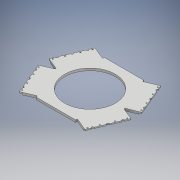
# Autodesk Inventor part: topplate change axes
Saved by Autodesk Inventor 2018 (Build 220112000, 112)
## iProperties
Created: 2018-06-04
Part Number: topplate change axes
Material: Generic
Document SubType Name: Modeling
Designer: John Viljoen
Density: 1 g/cm^3
Appearance: Default
Author: John Viljoen
Autodesk Inventor part; units mm, degrees
ref_plane "YZ Plane" through (0, 0, 0) normal (1, 0, 0) x (0, 1, 0)
ref_plane "XZ Plane" through (0, 0, 0) normal (0, 1, 0) x (-1, 0, 0)
ref_plane "XY Plane" through (0, 0, 0) normal (0, 0, 1) x (1, 0, 0)
sketch "Sketch1" plane through (0, 0, 0) normal (0, 0, 1) x (1, 0, 0)
  line L0 (0, 5) -> (0, 0)
  line L1 (0, 0) -> (109.5, 0)
  line L2 (109.5, 0) -> (109.5, 5)
  line L3 (109.5, 5) -> (145.4775, -9.976)
  line L4 (145.4775, -9.976) -> (150.4727, 2.0242)
  arc A0 (152.913, 7.8866) -> (150.4727, 2.0242) centre (151.6928, 4.9554) ccw
  line L5 (152.913, 7.8866) -> (162.9034, 31.887)
  arc A1 (165.3436, 37.7494) -> (162.9034, 31.887) centre (164.1235, 34.8182) ccw
  line L6 (165.3436, 37.7494) -> (175.334, 61.7498)
  arc A2 (177.7743, 67.6121) -> (175.334, 61.7498) centre (176.5542, 64.6809) ccw
  line L7 (177.7743, 67.6121) -> (182.7695, 79.6123)
  line L8 (182.7695, 79.6123) -> (146.792, 94.5883)
  line L9 (146.792, 94.5883) -> (182.7695, 109.5643)
  line L10 (182.7695, 109.5643) -> (177.7743, 121.5645)
  arc A3 (175.334, 127.4269) -> (177.7743, 121.5645) centre (176.5542, 124.4957) ccw
  line L11 (175.334, 127.4269) -> (165.3436, 151.4273)
  arc A4 (162.9034, 157.2897) -> (165.3436, 151.4273) centre (164.1235, 154.3585) ccw
  line L12 (162.9034, 157.2897) -> (152.913, 181.29)
  arc A5 (150.4727, 187.1524) -> (152.913, 181.29) centre (151.6928, 184.2212) ccw
  line L13 (150.4727, 187.1524) -> (145.4775, 199.1526)
  line L14 (145.4775, 199.1526) -> (109.5, 184.1766)
  line L15 (109.5, 184.1766) -> (109.5, 189.1766)
  line L16 (109.5, 189.1766) -> (0, 189.1766)
  line L17 (0, 189.1766) -> (0, 184.1766)
  line L18 (0, 184.1766) -> (-35.9775, 199.1526)
  line L19 (-35.9775, 199.1526) -> (-40.9727, 187.1524)
  arc A6 (-43.413, 181.29) -> (-40.9727, 187.1524) centre (-42.1928, 184.2212) ccw
  line L20 (-43.413, 181.29) -> (-53.4034, 157.2897)
  arc A7 (-55.8436, 151.4273) -> (-53.4034, 157.2897) centre (-54.6235, 154.3585) ccw
  line L21 (-55.8436, 151.4273) -> (-65.834, 127.4269)
  arc A8 (-68.2743, 121.5645) -> (-65.834, 127.4269) centre (-67.0542, 124.4957) ccw
  line L22 (-68.2743, 121.5645) -> (-73.2695, 109.5643)
  line L23 (-73.2695, 109.5643) -> (-37.292, 94.5883)
  line L24 (-37.292, 94.5883) -> (-73.2695, 79.6123)
  line L25 (-73.2695, 79.6123) -> (-68.2743, 67.6121)
  arc A9 (-65.834, 61.7498) -> (-68.2743, 67.6121) centre (-67.0542, 64.6809) ccw
  line L26 (-65.834, 61.7498) -> (-55.8436, 37.7494)
  arc A10 (-53.4034, 31.887) -> (-55.8436, 37.7494) centre (-54.6235, 34.8182) ccw
  line L27 (-53.4034, 31.887) -> (-43.413, 7.8866)
  arc A11 (-40.9727, 2.0242) -> (-43.413, 7.8866) centre (-42.1928, 4.9554) ccw
  line L28 (-40.9727, 2.0242) -> (-35.9775, -9.976)
  line L29 (-35.9775, -9.976) -> (0, 5)
  circle A12 centre (-35.5423, -2.7596) radius 1.5
  circle A13 centre (54.75, 94.5883) radius 70
  circle A14 centre (154.973, 168.0663) radius 1.5
  circle A15 centre (-67.8404, 114.345) radius 1.5
  circle A16 centre (-57.907, 138.2085) radius 1.5
  circle A17 centre (-45.4757, 168.0728) radius 1.5
  circle A18 centre (-35.5423, 191.9362) radius 1.5
  circle A19 centre (145.0396, 191.9297) radius 1.5
  circle A20 centre (167.4043, 138.2019) radius 1.5
  circle A21 centre (177.3377, 114.3385) radius 1.5
  circle A22 centre (177.3404, 74.8316) radius 1.5
  circle A23 centre (167.407, 50.9682) radius 1.5
  circle A24 centre (154.9757, 21.1038) radius 1.5
  circle A25 centre (145.0423, -2.7596) radius 1.5
  circle A26 centre (-67.8404, 74.8316) radius 1.5
  circle A27 centre (-57.907, 50.9682) radius 1.5
  circle A28 centre (-45.4757, 21.1038) radius 1.5
  constraints: 60 end point, 29 centre point, 24 point on circle
extrude "Extrusion1" add sketch "Sketch1" along normal blind 6.35
sketch "Sketch2" plane through (-35.9775, 199.1526, 6.35) normal (0.3842953, 0.9232102, 0) x (0.9232102, -0.3842953, 0)
  line L0 (0, 6.35) -> (6.35, 6.35)
  line L1 (6.35, 6.35) -> (6.35, 3.175)
  line L2 (6.35, 3.175) -> (0, 3.175)
  line L3 (0, 3.175) -> (0, 6.35)
  point P0 (109.7482, 6.35)
  dimension "d2" = 6.35
  constraints: 8 end point, 2 parallel, 1 horizontal, 1 perpendicular
  measures "d2" distance of L1.end L2.end
extrude "Extrusion2" cut sketch "Sketch2" against normal through all
sketch "Sketch3" plane through (-73.2695, 79.6123, 6.35) normal (-0.3842953, 0.9232102, 0) x (0.9232102, 0.3842953, 0)
  line L0 (0, 6.35) -> (6.35, 6.35)
  line L1 (6.35, 6.35) -> (6.35, 3.175)
  line L2 (6.35, 3.175) -> (0, 3.175)
  line L3 (0, 3.175) -> (0, 6.35)
  point P0 (37.0485, 6.35)
  dimension "d5" = 6.35
  constraints: 8 end point, 2 parallel, 1 horizontal, 1 perpendicular
  measures "d5" distance of L1.end L2.end
extrude "Extrusion3" cut sketch "Sketch3" against normal through all
sketch "Sketch4" plane through (109.5, 184.1766, 6.35) normal (-0.3842953, 0.9232102, 0) x (0.9232102, 0.3842953, 0)
  line L0 (38.97, 6.35) -> (32.62, 6.35)
  line L1 (32.62, 6.35) -> (32.62, 3.175)
  line L2 (32.62, 3.175) -> (38.97, 3.175)
  line L3 (38.97, 3.175) -> (38.97, 6.35)
  point P0 (-171.8697, 6.35)
  dimension "d8" = 6.35
  constraints: 8 end point, 2 parallel, 1 horizontal, 1 perpendicular
  measures "d8" distance of L2.end L1.end
extrude "Extrusion4" cut sketch "Sketch4" against normal through all
sketch "Sketch5" plane through (146.792, 94.5883, 6.35) normal (0.3842953, 0.9232102, 0) x (0.9232102, -0.3842953, 0)
  line L0 (38.97, 6.35) -> (32.62, 6.35)
  line L1 (32.62, 6.35) -> (32.62, 3.175)
  line L2 (32.62, 3.175) -> (38.97, 3.175)
  line L3 (38.97, 3.175) -> (38.97, 6.35)
  point P0 (-99.17, 6.35)
  dimension "d11" = 6.35
  constraints: 8 end point, 2 parallel, 1 horizontal, 1 perpendicular
  measures "d11" distance of L2.end L1.end
extrude "Extrusion5" cut sketch "Sketch5" against normal through all
fillet "Fillet1" radius 2 6 edges at (109.5, 184.1766, 3.175) (0, 184.1766, 3.175) (-37.292, 94.5883, 3.175) (0, 5, 3.175) (109.5, 5, 3.175) (146.792, 94.5883, 3.175)
body "Solid1"
